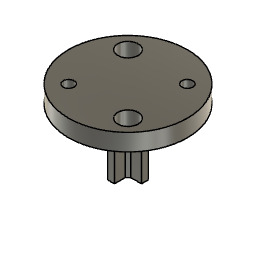
cross_peg (Autodesk Fusion 360 design; units mm, degrees)
Autodesk Fusion 360 part; units mm, degrees
sketch "Sketch1" plane through (0, 0, 0) normal (0, 0, 1) x (1, 0, 0)
  circle A0 centre (-17.5, -17.5) radius 3.25
  circle A1 centre (-17.5, 17.5) radius 3.25
  circle A2 centre (17.5, 17.5) radius 3.25
  circle A3 centre (17.5, -17.5) radius 3.25
  circle A4 centre (0, 0) radius 35
  circle A5 centre (-17.5, 17.5) radius 6
  circle A6 centre (17.5, -17.5) radius 6
  dimension "d2" = 360
  dimension "d3" = 70
  dimension "d4" = 17.5
  dimension "d5" = 17.5
  dimension "d6" = 6.5
  dimension "d23" = 12
  dimension "d24" = 12
  constraint coincident A4.centre origin
  constraint concentric A1 A5
  constraint concentric A3 A6
  measures "d3" diameter of A4
  measures "d4" vertical distance of A4.centre A2.centre
  measures "d5" horizontal distance of A4.centre A2.centre
  measures "d6" diameter of A2
  measures "d23" diameter of A5
  measures "d24" diameter of A6
extrude "Extrude1" add sketch "Sketch1" against normal blind 10 contours A4 | A5 | A6 makes body 1
sketch "Sketch6" plane through (0, 0, 0) normal (0, 0, 1) x (-1, 0, 0)
  circle A0 centre (17.5, 17.5) radius 3.25
  circle A1 centre (17.5, -17.5) radius 3.25
  circle A2 centre (-17.5, -17.5) radius 3.25
  circle A3 centre (-17.5, 17.5) radius 3.25
  circle A4 centre (0, 0) radius 35
  circle A5 centre (17.5, 17.5) radius 6
  circle A6 centre (-17.5, -17.5) radius 6
  dimension "d26" = 12
  dimension "d27" = 12
  constraint concentric A0 A5
  constraint concentric A2 A6
  measures "d26" diameter of A5
  measures "d27" diameter of A6
extrude "Extrude6" cut sketch "Sketch6" against normal blind 10 contours A5 | A6 bodies 1
sketch "Sketch2" plane through (0, 0, 0) normal (0, 0, 1) x (-1, 0, 0)
  circle A0 centre (17.5, -17.5) radius 3.25
  circle A1 centre (-17.5, 17.5) radius 3.25
  circle A2 centre (0, 0) radius 35
  line L0 (-10, 10) -> (10, 10)
  line L1 (10, 10) -> (10, -10)
  line L2 (10, -10) -> (-10, -10)
  line L3 (-10, -10) -> (-10, 10)
  line L4 (-10, 10) -> (10, -10) construction
  line L5 (10, 10) -> (-10, -10) construction
  circle A3 centre (-17.5, -17.5) radius 6
  circle A4 centre (17.5, 17.5) radius 6
  dimension "d9" = 20
  dimension "d10" = 20
  constraint horizontal L0
  constraint perpendicular L0 L1
  constraint parallel L0 L2
  constraint parallel L1 L3
  constraint coincident L4 A2.centre
  constraint coincident L5 A2.centre
  constraint coincident A2.centre origin
  measures "d9" distance of L0.end L1.end
  measures "d10" distance of L1.end L2.end
extrude "Extrude2" add sketch "Sketch2" along normal blind 10 separate body contours L0 L1 L2 L3 makes body 2
sketch "Sketch3" plane through (0, 0, 10) normal (0, 0, 1) x (-1, 0, 0)
  line L0 (-10, -10) -> (10, -10)
  line L1 (10, -10) -> (10, 10)
  line L2 (10, 10) -> (-10, 10)
  line L3 (-10, 10) -> (-10, -10)
  line L4 (-2.02, -10) -> (2.02, -10)
  line L5 (2.02, -10) -> (2.02, 10)
  line L6 (2.02, 10) -> (-2.02, 10)
  line L7 (-2.02, 10) -> (-2.02, -10)
  line L8 (-2.02, -10) -> (2.02, 10) construction
  line L9 (2.02, -10) -> (-2.02, 10) construction
  dimension "d13" = 4.04
  dimension "d14" = 20
  constraint horizontal L4
  constraint perpendicular L4 L5
  constraint parallel L4 L6
  constraint parallel L5 L7
  constraint coincident L8 origin
  constraint coincident L9 origin
  measures "d13" distance of L5.end L6.end
  measures "d14" distance of L4.end L5.end
extrude "Extrude3" add sketch "Sketch3" along normal blind 25 separate body contours L0 L2 L4 L5 L6 L7 makes body 3
sketch "Sketch4" plane through (0, 0, 10) normal (0, 0, 1) x (-1, 0, 0)
  line L0 (-10, -10) -> (10, -10)
  line L1 (10, -10) -> (10, 10)
  line L2 (10, 10) -> (-10, 10)
  line L3 (-10, 10) -> (-10, -10)
  line L4 (2.02, 2.02) -> (10, 2.02)
  line L5 (10, 2.02) -> (10, -2.02)
  line L6 (10, -2.02) -> (2.02, -2.02)
  line L7 (2.02, -2.02) -> (2.02, 2.02)
  line L8 (0, 0) -> (12.844, 0) construction
  line L9 (2.02, -10) -> (2.02, 10)
  dimension "d22" = 4.04
  constraint horizontal L4
  constraint vertical L5
  constraint horizontal L6
  constraint vertical L7
  constraint coincident L1 L5.end
  constraint coincident L8.start origin
  constraint perpendicular L5 L8
  constraint symmetric L4 L6 L8
  constraint coincident L4.start L9
  measures "d22" distance of L4 L6
extrude "Extrude4" add sketch "Sketch4" along normal blind 25 separate body contours L1 L4 L5 L6 L7 L9 makes body 4
sketch "Sketch5" plane through (0, 0, 10) normal (0, 0, 1) x (-1, 0, 0)
  line L0 (-10, -10) -> (10, -10)
  line L1 (10, -10) -> (10, 10)
  line L2 (10, 10) -> (-10, 10)
  line L3 (-10, 10) -> (-10, -10)
  line L4 (-2.02, 2.02) -> (-10, 2.02)
  line L5 (-10, 2.02) -> (-10, -2.02)
  line L6 (-10, -2.02) -> (-2.02, -2.02)
  line L7 (-2.02, -2.02) -> (-2.02, 2.02)
  line L8 (0, 0) -> (-12.3958, 0) construction
  line L9 (-2.02, 10) -> (-2.02, -10)
  dimension "d19" = 4.04
  constraint horizontal L4
  constraint vertical L5
  constraint horizontal L6
  constraint vertical L7
  constraint coincident L3 L5.end
  constraint coincident L8.start origin
  constraint perpendicular L3 L8
  constraint symmetric L4 L6 L8
  constraint coincident L4.start L9
  measures "d19" distance of L4.end L5.end
extrude "Extrude5" add sketch "Sketch5" along normal blind 25 separate body contours L3 L4 L5 L6 L7 L9 makes body 5
sketch "Sketch7" plane through (0, 0, 10) normal (0, 0, 1) x (-1, 0, 0)
  line L0 (-10, -10) -> (10, -10)
  line L1 (10, -10) -> (10, 10)
  line L2 (10, 10) -> (-10, 10)
  line L3 (-10, 10) -> (-10, -10)
  line L4 (3.66, 2.02) -> (2.02, 2.02)
  line L5 (2.02, 2.02) -> (2.02, 3.66)
  line L6 (2.02, -10) -> (2.02, 10)
  line L7 (10, 2.02) -> (2.02, 2.02)
  line L8 (3.66, 2.02) -> (2.02, 3.66)
  dimension "d30" = 1.64
  dimension "d31" = 1.64
  constraint horizontal L4
  constraint perpendicular L4 L5
  constraint coincident L4.end L6
  constraint coincident L4.end L7
  measures "d30" distance of L4.start L4.end
  measures "d31" distance of L4.end L5.end
extrude "Extrude7" add sketch "Sketch7" along normal blind 25 separate body contours L4 L5 L6 L7 L8 makes body 6
mirror "Mirror1" about plane through (0, 0, 0) normal (1, 0, 0) of bodies 6 makes body 7
mirror "Mirror2" about plane through (0, 0, 0) normal (0, 1, 0) of bodies 7 makes body 8
mirror "Mirror3" about plane through (0, 0, 0) normal (1, 0, 0) of bodies 8 makes body 9
move_body "Move1" bodies 4 7 6 2 1 5 3 9 8 to x (1, 0, 0) y (0, -1, 0) z (0, 0, -1) at (0, 0, 0)
move_body "Move2" bodies 3 4 7 5 8 6 2 9 1 to x (1, 0, 0) y (0, 1, 0) z (0, 0, 1) at (0, 0, 10)
